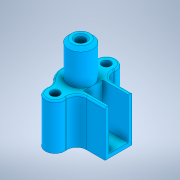
# Autodesk Inventor part: caster-bng
Saved by Autodesk Inventor 2020 (Build 240168000, 168)
## iProperties
Created: 2020-11-05
Part Number: caster-bng
Material: Generic
Document SubType Name: Modeling
Designer: alnwlsn
Density: 1 g/cm^3
Appearance: Default
Author: alnwlsn
Autodesk Inventor part; units mm, degrees
ref_plane "YZ Plane" through (0, 0, 0) normal (1, 0, 0) x (0, 1, 0)
ref_plane "XZ Plane" through (0, 0, 0) normal (0, 1, 0) x (-1, 0, 0)
ref_plane "XY Plane" through (0, 0, 0) normal (0, 0, 1) x (1, 0, 0)
sketch "Sketch1" plane through (0, 0, 0) normal (0, 0, 1) x (1, 0, 0)
  line L0 (0, 0) -> (0, 38.4841) construction
  line L1 (2.8, 25) -> (3.8, 24)
  line L2 (3.8, 24) -> (3.8, 0)
  line L3 (2.8, 25) -> (1.4, 25)
  line L4 (1.4, 25) -> (1.4, 0)
  line L5 (1.4, 0) -> (3.8, 0)
  dimension "d1" = 1.4
  dimension "d8" = 1
  dimension "d20" = 3.8
  constraints: 12 end point, 2 horizontal, 1 perpendicular, 1 point on line, 1 vertical
  measures "d1" distance between parallel lines of L0 L4
  measures "d8" horizontal distance of L1.end L1.start
  measures "d20" distance between parallel lines of L2 L0
revolve "Revolution1" add sketch "Sketch1" angle 360 about axis through (0, 0, 0) along (0, 1, 0)
chamfer "Chamfer1" distance 0.5 angle 45 2 edges at (-1.4, 25, 0) (-1.4, 0, 0)
sketch "Sketch6" plane through (0, 0, 0) normal (0, -1, 0) x (1, 0, 0)
  line L0 (0, 0) -> (0, -8) construction
  circle A0 centre (0, 8) radius 3
  circle A1 centre (0, -8) radius 3
  circle A2 centre (0, 0) radius 6
  line L1 (0, 0) -> (0, 8) construction
  circle A3 centre (0, 8) radius 1.35
  circle A4 centre (0, -8) radius 1.35
  circle A5 centre (0, 0) radius 1.9 projected
  line L2 (11.8, 4.2) -> (2, 4.2)
  line L3 (2, 4.2) -> (2, -4.2)
  line L4 (2, -4.2) -> (11.8, -4.2)
  line L5 (11.8, -4.2) -> (11.8, 4.2)
  line L6 (0, 0) -> (2, 4.2) construction
  line L7 (0, 0) -> (2, -4.2) construction
  point P0 (1.9111, -5.6875)
  point P1 (1.9111, 5.6875)
  point P2 (-1.9111, 5.6875)
  point P3 (-1.9111, -5.6875)
  point P4 (4.2849, 4.2)
  point P5 (4.2849, -4.2)
  dimension "d24" = 6
  dimension "d26" = 8
  dimension "d27" = 12
  dimension "d28" = 2.7
  dimension "d33" = 2
  dimension "d34" = 8.4
  dimension "d35" = 11.8
  constraints: 16 end point, 6 coincident, 5 centre point, 2 equal length, 2 equal radius, 2 parallel, 2 vertical, 1 horizontal, 1 perpendicular
  measures "d24" diameter of A1
  measures "d26" distance of L1.start L1.end
  measures "d27" diameter of A2
  measures "d28" diameter of A4
  measures "d33" horizontal distance of L6.start L2.end
  measures "d34" distance of L4.end L2.start
  measures "d35" distance from line of L5 point (0, 0)
extrude "Extrusion3" add sketch "Sketch6" against normal blind 14.2
fillet "Fillet1" radius 4 4 edges at (1.9111, 7.1, 5.6875) (-1.9111, 7.1, -5.6875) (1.9111, 7.1, -5.6875) (-1.9111, 7.1, 5.6875)
sketch "Sketch7" plane through (0, 0, -8) normal (0, -1, 0) x (1, 0, 0)
  circle A0 centre (0, 8) radius 6
  constraints: 1 centre point, 1 coincident
sketch "Sketch8" plane through (0, 0, 8) normal (0, -1, 0) x (1, 0, 0)
  point P0 (0, -8)
sketch "Sketch10" plane through (11.8, 0, 4.2) normal (1, 0, 0) x (0, 0, -1)
  line L0 (7.2, 1.2) -> (1.2, 1.2)
  line L1 (1.2, 1.2) -> (1.2, 14.2)
  line L2 (1.2, 14.2) -> (7.2, 14.2)
  line L3 (7.2, 14.2) -> (7.2, 1.2)
  line L4 (7.2, 1.2) -> (4.2, 0) construction
  line L5 (4.2, 0) -> (1.2, 1.2) construction
  line L6 (8.4, 0) -> (0, 0) projected
  dimension "d39" = 6
  dimension "d40" = 1.2
  dimension "d41" = 13
  constraints: 12 end point, 2 parallel, 1 equal length, 1 horizontal, 1 perpendicular
  measures "d39" distance of L0.start L0.end
  measures "d40" distance between parallel lines of L6 L0
  measures "d41" distance of L0.end L1.end
extrude "Extrusion4" cut sketch "Sketch10" against normal blind 8
fillet "Fillet4" radius 3 2 edges at (4.2849, 7.1, 4.2) (4.2849, 7.1, -4.2)
fillet "Fillet5" radius 0.5 11 edges at (-3.1855, 14.2, -5.8429) (-6, 14.2, 0) (-3.1855, 14.2, 5.8429) (0, 14.2, 11) (2.961, 14.2, 7.446) (3.8182, 14.2, 5.092) (8.8764, 14.2, 4.2) (2.961, 14.2, -7.446) (3.8182, 14.2, -5.092) (8.8764, 14.2, -4.2) (0, 14.2, -11)
body "Solid1"
